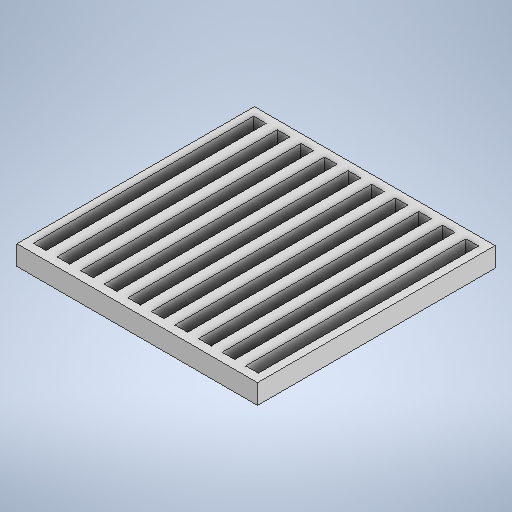
# Autodesk Inventor part: DisplayModuleHousingCap
Saved by Autodesk Inventor 2025.1 (Build 291241020, 241B)
## iProperties
Created: 2024-10-14
Part Number: DisplayModuleHousingCap
Material: Generic
Document SubType Name: Modeling
Designer: Si Teng Wu
Density: 1 g/cm^3
Appearance: Default
Author: Si Teng Wu
Autodesk Inventor part; units mm, degrees
ref_plane "YZ Plane" through (0, 0, 0) normal (1, 0, 0) x (0, 1, 0)
ref_plane "XZ Plane" through (0, 0, 0) normal (0, 1, 0) x (-1, 0, 0)
ref_plane "XY Plane" through (0, 0, 0) normal (0, 0, 1) x (1, 0, 0)
sketch "Sketch1" plane through (0, 0, 0) normal (0, 1, 0) x (-1, 0, 0)
  line L0 (28.6, -28) -> (25.4, -28)
  line L1 (25.4, -28) -> (25.4, 28)
  line L2 (25.4, 28) -> (28.6, 28)
  line L3 (28.6, 28) -> (28.6, -28)
  line L4 (28.6, -28) -> (25.4, 28) construction
  line L5 (25.4, -28) -> (28.6, 28) construction
  line L6 (22.6, -28) -> (19.4, -28)
  line L7 (19.4, -28) -> (19.4, 28)
  line L8 (19.4, 28) -> (22.6, 28)
  line L9 (22.6, 28) -> (22.6, -28)
  line L10 (22.6, -28) -> (19.4, 28) construction
  line L11 (19.4, -28) -> (22.6, 28) construction
  line L12 (16.6, -28) -> (13.4, -28)
  line L13 (13.4, -28) -> (13.4, 28)
  line L14 (13.4, 28) -> (16.6, 28)
  line L15 (16.6, 28) -> (16.6, -28)
  line L16 (16.6, -28) -> (13.4, 28) construction
  line L17 (13.4, -28) -> (16.6, 28) construction
  line L18 (10.6, -28) -> (7.4, -28)
  line L19 (7.4, 28) -> (10.6, 28)
  line L20 (7.4, -28) -> (7.4, 28)
  line L21 (10.6, -28) -> (7.4, 28) construction
  line L22 (7.4, -28) -> (10.6, 28) construction
  line L23 (10.6, 28) -> (10.6, -28)
  line L24 (4.6, -28) -> (1.4, -28)
  line L25 (1.4, 28) -> (4.6, 28)
  line L26 (1.4, -28) -> (1.4, 28)
  line L27 (4.6, -28) -> (1.4, 28) construction
  line L28 (1.4, -28) -> (4.6, 28) construction
  line L29 (4.6, 28) -> (4.6, -28)
  line L30 (-1.4, -28) -> (-4.6, -28)
  line L31 (-4.6, 28) -> (-1.4, 28)
  line L32 (-4.6, -28) -> (-4.6, 28)
  line L33 (-1.4, -28) -> (-4.6, 28) construction
  line L34 (-4.6, -28) -> (-1.4, 28) construction
  line L35 (-1.4, 28) -> (-1.4, -28)
  line L36 (-7.4, 28) -> (-7.4, -28)
  line L37 (-10.6, -28) -> (-7.4, 28) construction
  line L38 (-10.6, -28) -> (-10.6, 28)
  line L39 (-7.4, -28) -> (-10.6, 28) construction
  line L40 (-10.6, 28) -> (-7.4, 28)
  line L41 (-7.4, -28) -> (-10.6, -28)
  line L42 (-13.4, 28) -> (-13.4, -28)
  line L43 (-16.6, -28) -> (-13.4, 28) construction
  line L44 (-16.6, -28) -> (-16.6, 28)
  line L45 (-13.4, -28) -> (-16.6, 28) construction
  line L46 (-16.6, 28) -> (-13.4, 28)
  line L47 (-13.4, -28) -> (-16.6, -28)
  line L48 (-19.4, 28) -> (-19.4, -28)
  line L49 (-22.6, -28) -> (-19.4, 28) construction
  line L50 (-22.6, -28) -> (-22.6, 28)
  line L51 (-19.4, -28) -> (-22.6, 28) construction
  line L52 (-22.6, 28) -> (-19.4, 28)
  line L53 (-19.4, -28) -> (-22.6, -28)
  line L54 (-25.4, 28) -> (-25.4, -28)
  line L55 (-28.6, -28) -> (-25.4, 28) construction
  line L56 (-28.6, -28) -> (-28.6, 28)
  line L57 (-25.4, -28) -> (-28.6, 28) construction
  line L58 (-28.6, 28) -> (-25.4, 28)
  line L59 (-25.4, -28) -> (-28.6, -28)
  line L60 (0, 0) -> (33.435, 0)
  point P0 (27, 28)
  point P1 (21, 28)
  point P2 (15, 28)
  point P3 (9, 28)
  point P4 (3, 28)
  point P5 (-3, 28)
  point P6 (-9, 28)
  point P7 (-15, 28)
  point P8 (-21, 28)
  point P9 (-27, 28)
  point P10 (27, -28)
  point P11 (21, 0)
  point P12 (27, 0)
  point P13 (15, 0)
  point P14 (21, 0)
  point P15 (9, 0)
  point P16 (15, 0)
  point P17 (3, 0)
  point P18 (9, 0)
  point P19 (-3, 0)
  point P20 (3, 0)
  point P21 (-9, 0)
  point P22 (-3, 0)
  point P23 (-15, 0)
  point P24 (-9, 0)
  point P25 (-21, 0)
  point P26 (-15, 0)
  point P27 (-27, 0)
  point P28 (-21, 0)
  point P29 (27, 0)
  dimension "d0" = 3.2
  dimension "d1" = 3.2
  dimension "d2" = 3.2
  dimension "d3" = 3.2
  dimension "d4" = 3.2
  dimension "d5" = 3.2
  dimension "d6" = 3.2
  dimension "d7" = 3.2
  dimension "d8" = 3.2
  dimension "d9" = 6
  dimension "d10" = 6
  dimension "d11" = 6
  dimension "d12" = 6
  dimension "d13" = 6
  dimension "d14" = 6
  dimension "d15" = 6
  dimension "d16" = 6
  dimension "d17" = 6
  dimension "d19" = 3
  dimension "d26" = 56
  constraints: 122 end point, 30 midpoint, 20 parallel, 19 collinear, 11 horizontal, 10 perpendicular, 1 horizontal alignment, 1 other
  measures "d0" distance between parallel lines of L1 L3
  measures "d1" distance between parallel lines of L13 L15
  measures "d2" distance between parallel lines of L20 L23
  measures "d3" distance between parallel lines of L26 L29
  measures "d4" distance between parallel lines of L32 L35
  measures "d5" distance between parallel lines of L38 L36
  measures "d6" distance between parallel lines of L44 L42
  measures "d7" distance between parallel lines of L50 L48
  measures "d8" distance between parallel lines of L56 L54
  measures "d9" distance of point (21, 0) point (27, 0)
  measures "d10" distance of point (15, 0) point (21, 0)
  measures "d11" distance of point (9, 0) point (15, 0)
  measures "d12" distance of point (3, 0) point (9, 0)
  measures "d13" distance of point (-3, 0) point (3, 0)
  measures "d14" distance of point (-9, 0) point (-3, 0)
  measures "d15" distance of point (-15, 0) point (-9, 0)
  measures "d16" distance of point (-21, 0) point (-15, 0)
  measures "d17" distance of point (-27, 0) point (-21, 0)
  measures "d19" distance of point (-3, 0) L60.start
  measures "d26" distance between parallel lines of L2 L0
sketch "Sketch2" plane through (0, 0, 0) normal (0, 1, 0) x (-1, 0, 0)
  line L0 (-30.6, -30.2) -> (30.6, -30.2)
  line L1 (30.6, -30.2) -> (30.6, 30.2)
  line L2 (30.6, 30.2) -> (-30.6, 30.2)
  line L3 (-30.6, 30.2) -> (-30.6, -30.2)
  line L4 (-30.6, -30.2) -> (30.6, 30.2) construction
  line L5 (30.6, -30.2) -> (-30.6, 30.2) construction
  point P0 (0, 0)
  dimension "d20" = 60.4
  dimension "d21" = 61.2
  constraints: 12 end point, 2 midpoint, 2 parallel, 1 horizontal, 1 perpendicular
  measures "d20" distance of L0.end L1.end
  measures "d21" distance of L0.start L0.end
extrude "Extrusion1" add sketch "Sketch2" against normal blind 5
extrude "Extrusion2" cut sketch "Sketch1" against normal blind 3.5
equation "\"d1\" = d0"
equation "\"d2\" = d0"
equation "\"d3\" = d0"
equation "\"d4\" = d0"
equation "\"d5\" = d4"
equation "\"d6\" = d5"
equation "\"d7\" = d6"
equation "\"d8\" = d6"
equation "\"d10\" = d9"
equation "\"d11\" = d10"
equation "\"d12\" = d11"
equation "\"d13\" = d12"
equation "\"d14\" = d13"
equation "\"d15\" = d14"
equation "\"d16\" = d15"
equation "\"d17\" = d16"
equation "\"d19\" = 0.5 * d13"
body "Solid1"
